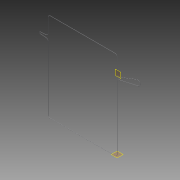
# Autodesk Inventor part: STRING BED
Saved by Autodesk Inventor 2013 (Build 170138000, 138)
## iProperties
Created: 2014-06-23
Part Number: STRING BED
Material: Generic
Document SubType Name: Modeling
Designer: employee
Density: 1 g/cm^3
Author: employee
Autodesk Inventor part; units mm, degrees
ref_plane "YZ Plane" through (0, 0, 0) normal (1, 0, 0) x (0, 1, 0)
ref_plane "XZ Plane" through (0, 0, 0) normal (0, 1, 0) x (-1, 0, 0)
ref_plane "Work Plane3" through (0, 0, -2.5) normal (0, 0, 1) x (1, 0, 0)
sketch "Sketch4" plane through (0, 0, -2.5) normal (0, 0, 1) x (1, 0, 0)
  circle A0 centre (5.25, 0) radius 8 construction
  circle A1 centre (5.25, -25) radius 8 construction
  arc A2 (-2.75, 42.5) -> (-10.75, 50.5) centre (-10.75, 42.5) ccw projected
  arc A3 (-248.75, 50.5) -> (-256.75, 42.5) centre (-248.75, 42.5) ccw projected
  arc A4 (-269.7437, -6.25) -> (-267.0357, 7.6665) centre (-264.75, 0) ccw construction
  circle A5 centre (-284.75, -12.5) radius 3.125 construction
  arc A6 (-267.0357, -32.6665) -> (-269.7437, -18.75) centre (-264.75, -25) ccw construction
  circle A7 centre (72.465, 7.5) radius 9 construction
  arc A8 (-10.75, -275.5) -> (-2.75, -267.5) centre (-10.75, -267.5) ccw projected
  arc A9 (-256.75, -267.5) -> (-248.75, -275.5) centre (-248.75, -267.5) ccw projected
  arc A10 (74.4805, -1.7837) -> (69.0044, 16.3473) centre (72.465, 7.5) ccw
  line L0 (69.0044, 16.3473) -> (8.1642, -7.4503)
  line L1 (74.4805, -1.7837) -> (3.5527, -17.1821)
  arc A11 (-2.75, 0) -> (8.1642, -7.4503) centre (5.25, 0) ccw
  line L2 (-2.75, 0) -> (-2.75, 42.5)
  line L3 (-10.75, 50.5) -> (-248.75, 50.5)
  line L4 (-256.75, 42.5) -> (-256.75, 0)
  arc A12 (-264.2113, -7.9818) -> (-256.75, 0) centre (-264.75, 0) ccw
  line L5 (-264.2113, -7.9818) -> (-284.9604, -9.3821)
  arc A13 (-284.9604, -9.3821) -> (-284.9604, -15.6179) centre (-284.75, -12.5) ccw
  line L6 (-284.9604, -15.6179) -> (-264.2113, -17.0182)
  arc A14 (-256.75, -25) -> (-264.2113, -17.0182) centre (-264.75, -25) ccw
  line L7 (-256.75, -25) -> (-256.75, -267.5)
  line L8 (-248.75, -275.5) -> (-10.75, -275.5)
  line L9 (-2.75, -267.5) -> (-2.75, -25)
  arc A15 (3.5527, -17.1821) -> (-2.75, -25) centre (5.25, -25) ccw
  point P0 (0, 0)
  dimension "d6" = 0.5
  constraints: 27 tangent, 22 point on circle, 20 end point, 6 centre point, 5 concentric, 2 perpendicular, 1 collinear, 1 vertical
  measures "d6" radial gap between concentric circles of A7 A10
ref_plane "Work Plane4" through (-2.75, -267.5, -2.5) normal (0, 1, 0) x (-1, 0, 0)
sketch "Sketch5" plane through (-2.75, -267.5, -2.5) normal (0, 1, 0) x (-1, 0, 0)
  circle A0 centre (0, 0) radius 0.5
  point P0 (-2.75, 2.5)
  dimension "d7" = 1
  constraints: 1 centre point, 1 coincident
  measures "d7" diameter of A0
sweep "Sweep1" add profiles "Sketch5" path "Sketch4"
body "Solid1"
